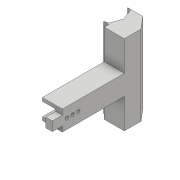
# Autodesk Inventor part: 32mm_x_120mm
Saved by Autodesk Inventor 2017 (Build 210142000, 142)
## iProperties
Created: 2018-04-21
Part Number: 32mm_x_120mm
Material: Generic
Document SubType Name: Modeling
Designer: Jeyy
Density: 1 g/cm^3
Appearance: Default
Author: Jeyy
Autodesk Inventor part; units mm, degrees
ref_plane "YZ Plane" through (0, 0, 0) normal (1, 0, 0) x (0, 1, 0)
ref_plane "XZ Plane" through (0, 0, 0) normal (0, 1, 0) x (-1, 0, 0)
sketch "Sketch1" plane through (0, 0, 0) normal (0, 0, 1) x (1, 0, 0)
  line L0 (0, 0) -> (25, 0)
  line L1 (25, 0) -> (25, 40)
  line L2 (25, 40) -> (0, 40)
  line L3 (0, 40) -> (0, 0)
  dimension "d1" = 25
  dimension "d2" = 40
  dimension "d3" = 25
  constraints: 8 end point, 2 perpendicular, 1 horizontal
  measures "d1" distance of L0.start L0.end
  measures "d2" distance of L0.end L1.end
  measures "d3" distance of L1.end L2.end
extrude "Extrusion1" add sketch "Sketch1" against normal blind 30
sketch "Sketch2" plane through (25, 0, 0) normal (1, 0, 0) x (0, 0, -1)
  line L0 (0, 0) -> (30, 0) projected
  circle A0 centre (15, 6.56) radius 2.46
  constraints: 1 centre point
extrude "Extrusion2" cut sketch "Sketch2" against normal blind 30
sketch "Sketch3" plane through (0, 0, 0) normal (-1, 0, 0) x (0, 0, 1)
  line L0 (0, 0) -> (-30, 0) projected
  line L1 (-25.05, 0) -> (-4.95, 0)
  line L2 (-4.95, 0) -> (-4.95, 33.12)
  line L3 (-4.95, 33.12) -> (-25.05, 33.12)
  line L4 (-25.05, 33.12) -> (-25.05, 0)
  dimension "d11" = 20.1
  constraints: 8 end point, 2 parallel, 1 perpendicular
  measures "d11" distance of L1.start L1.end
extrude "Extrusion3" cut sketch "Sketch3" against normal blind 20
sketch "Sketch4" plane through (0, 0, 0) normal (0, -1, 0) x (1, 0, 0)
  line L0 (20, -4.95) -> (20, -25.05) projected
  line L1 (20, -15) -> (25, -15)
  line L2 (25, 0) -> (25, -30) projected
  line L3 (20, -8.025) -> (25, -8.025)
  line L4 (25, -8.025) -> (25, -21.975)
  line L5 (25, -21.975) -> (20, -21.975)
  line L6 (20, -21.975) -> (20, -8.025)
  line L7 (20, -8.025) -> (25, -21.975) construction
  line L8 (25, -8.025) -> (20, -21.975) construction
  line L9 (25, -12.54) -> (25, -17.46) projected
  point P0 (0, 0)
  point P1 (22.5, -15)
  dimension "d14" = 13.95
  constraints: 14 end point, 5 midpoint, 2 parallel, 2 perpendicular
  measures "d14" distance of L3.end L4.end
extrude "Extrusion4" add sketch "Sketch4" along normal blind 15
sketch "Sketch5" plane through (20, 0, 0) normal (-1, 0, 0) x (0, 0, 1)
  circle A0 centre (-15, 6.56) radius 2.46 projected
  circle A1 centre (-15, 6.56) radius 4.7025
  circle A2 centre (-15, 6.56) radius 2.46 projected
  circle A3 centre (-15, 6.56) radius 2.46
  point P0 (0, 0)
  dimension "d17" = 9.405
  constraints: 2 centre point, 2 coincident
  measures "d17" diameter of A1
extrude "Extrusion5" cut sketch "Sketch5" against normal blind 2.1
sketch "Sketch6" plane through (25, 0, 0) normal (1, 0, 0) x (0, 0, -1)
  circle A0 centre (15, 6.56) radius 4.7025 projected
  line L0 (15, 6.56) -> (15, 23.56)
  circle A1 centre (15, 23.56) radius 2.46
  point P0 (0, 0)
  dimension "d20" = 17
  dimension "d21" = 4.92
  constraints: 2 end point, 1 centre point, 1 coincident, 1 vertical
  measures "d20" distance of L0.start L0.end
  measures "d21" diameter of A1
extrude "Extrusion6" cut sketch "Sketch6" against normal blind 10 contours A1
sketch "Sketch7" plane through (20, 0, 0) normal (-1, 0, 0) x (0, 0, 1)
  circle A0 centre (-15, 23.56) radius 2.46 projected
  circle A1 centre (-15, 23.56) radius 4.7025
  point P0 (0, 0)
  dimension "d24" = 9.405
  constraints: 1 centre point, 1 coincident
  measures "d24" diameter of A1
extrude "Extrusion7" cut sketch "Sketch7" against normal blind 2.1
sketch "Sketch9" plane through (25, 0, 0) normal (1, 0, 0) x (0, 0, -1)
  circle A0 centre (15, 6.56) radius 2.46 projected
  circle A1 centre (15, 6.56) radius 2.46
  circle A2 centre (15, 23.56) radius 2.46 projected
  circle A3 centre (15, 23.56) radius 2.46
  line L0 (30, 40) -> (30, 0) projected
  line L1 (30, 0) -> (30, 40)
  line L2 (30, 40) -> (0, 40)
  line L3 (0, 40) -> (0, 0)
  line L4 (0, 0) -> (8.025, 0) projected
  line L5 (21.975, 0) -> (21.975, -15)
  line L6 (21.975, -15) -> (8.025, -15)
  line L7 (8.025, -15) -> (8.025, 0)
  line L8 (0, 0) -> (8.025, 0)
  line L9 (21.975, 0) -> (30, 0)
  constraints: 16 end point, 4 parallel, 2 centre point, 2 coincident, 2 horizontal, 2 perpendicular
extrude "Extrusion8" add sketch "Sketch9" along normal blind 5
sketch "Sketch10" plane through (0, 40, 0) normal (0, 1, 0) x (1, 0, 0)
  line L0 (0, 30) -> (30, 30) projected
  line L1 (30, 0) -> (0, 0) projected
  line L2 (0, 30) -> (30, 30)
  line L3 (30, 30) -> (30, 0)
  line L4 (30, 0) -> (0, 0)
  line L5 (0, 0) -> (0, 30)
  constraints: 8 end point, 2 parallel, 1 horizontal, 1 perpendicular
extrude "Extrusion9" add sketch "Sketch10" along normal blind 30
sketch "Sketch12" plane through (30, 0, 0) normal (1, 0, 0) x (0, 0, -1)
  circle A0 centre (15, 6.56) radius 2.46 projected
  line L0 (15, 6.56) -> (15, 15.06)
  circle A1 centre (15, 15.06) radius 2.525
  point P0 (0, 0)
  dimension "d31" = 8.5
  dimension "d33" = 5.05
  constraints: 2 end point, 1 centre point, 1 coincident, 1 vertical
  measures "d31" distance of L0.start L0.end
  measures "d33" diameter of A1
extrude "Extrusion10" cut sketch "Sketch12" against normal blind 30 contours A1
sketch "Sketch14" plane through (0, 0, 0) normal (0, 0, 1) x (1, 0, 0)
  line L0 (30, 70) -> (0, 70) projected
  line L1 (0, 100) -> (-8, 100)
  line L2 (30, 0) -> (30, 70) projected
  line L3 (30, 118) -> (30, 70)
  line L4 (30, 105) -> (30, 100)
  line L5 (-2, 134) -> (-8, 136)
  line L6 (-2, 134) -> (4, 118)
  line L7 (-2, 102) -> (-8, 100)
  line L8 (-2, 102) -> (4, 118)
  line L9 (0, 70) -> (30, 70) projected
  line L10 (0, 70) -> (0, 100)
  line L11 (15, 136) -> (30, 118)
  line L12 (-8, 136) -> (15, 136)
  point P0 (0, 0)
  dimension "d47" = 30
  constraints: 20 end point, 2 vertical, 1 horizontal, 1 perpendicular, 1 point on line
  measures "d47" distance of L1.start L0.end
extrude "Extrusion12" add sketch "Sketch14" against normal blind 30
sketch "Sketch15" plane through (0, 0, -25.05) normal (-1, 0, 0) x (0, 0, 1)
  line L0 (0, 33.12) -> (20.1, 33.12) projected
  line L1 (20.1, 33.12) -> (20.1, 0) projected
  line L2 (0, 33.12) -> (20.1, 33.12)
  line L3 (20.1, 33.12) -> (20.1, 31.1)
  line L4 (20.1, 31.1) -> (0, 31.1)
  line L5 (0, 31.1) -> (0, 33.12)
  point P0 (25.05, 0)
  dimension "d57" = 2.02
  constraints: 8 end point, 2 parallel, 1 horizontal, 1 perpendicular, 1 point on line
  measures "d57" distance of L2.end L3.end
extrude "Extrusion13" add sketch "Sketch15" against normal blind 20
sketch "Sketch23" plane through (0, 0, 0) normal (0, 0, 1) x (1, 0, 0)
  line L0 (0, 100) -> (-8, 100) projected
  line L1 (-8, 100) -> (-2, 102) projected
  line L2 (-8, 100) -> (-2, 102)
  line L3 (-2, 102) -> (4, 118) projected
  line L4 (-2, 102) -> (4, 118)
  line L5 (-2, 134) -> (4, 118) projected
  line L6 (4, 118) -> (-2, 134)
  line L7 (-2, 134) -> (-8, 136) projected
  line L8 (-2, 134) -> (-8, 136)
  line L9 (-8, 136) -> (15, 136) projected
  line L10 (-8, 136) -> (15, 136)
  line L11 (30, 118) -> (15, 136) projected
  line L12 (15, 136) -> (30, 118)
  line L13 (30, 118) -> (30, 93)
  line L14 (30, 0) -> (30, 118) projected
  line L15 (30, 93) -> (0, 93)
  line L16 (0, 93) -> (0, 100)
  line L17 (-8, 100) -> (0, 100)
  point P0 (0, 0)
  dimension "d85" = 25
  constraints: 20 end point, 7 collinear, 2 perpendicular, 1 point on line
  measures "d85" distance of L11.start L13.end
extrude "Extrusion14" add sketch "Sketch23" along normal blind 45
ref_plane "Work Plane1" through (0, 0, -15) normal (0, 0, 1) x (1, 0, 0)
mirror "Mirror1" about plane through (0, 0, -15) normal (0, 0, 1) of "Extrusion14"
body "Solid1"
